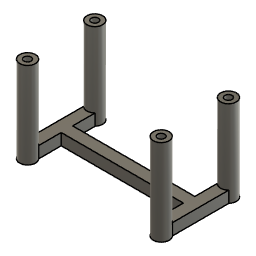
bracketEspHouse (Autodesk Fusion 360 design; units mm, degrees)
Autodesk Fusion 360 part; units mm, degrees
sketch "Schizzo8" plane through (0, 0, 0) normal (0, 1, 0) x (1, 0, 0)
  line L0 (45.3365, 90.3085) -> (91.8565, 90.3085)
  line L1 (91.8565, 90.3085) -> (91.8565, 66.9085)
  line L2 (91.8565, 66.9085) -> (45.3365, 66.9085)
  line L3 (45.3365, 66.9085) -> (45.3365, 90.3085)
  circle A0 centre (45.3365, 90.3085) radius 2.75
  circle A1 centre (91.8565, 90.3085) radius 2.75
  circle A2 centre (91.8565, 66.9085) radius 2.75
  circle A3 centre (45.3365, 66.9085) radius 2.75
  line L4 (45.3365, 90.3085) -> (47.3365, 90.3085)
  line L5 (45.3365, 90.3085) -> (43.3365, 90.3085)
  line L6 (43.3365, 90.3085) -> (43.3365, 66.9085)
  line L7 (47.3365, 90.3085) -> (47.3365, 66.9085)
  line L8 (91.8565, 90.3085) -> (93.8565, 90.3085)
  line L9 (91.8565, 90.3085) -> (89.8565, 90.3085)
  line L10 (89.8565, 90.3085) -> (89.8565, 66.9085)
  line L11 (93.8565, 90.3085) -> (93.8565, 66.9085)
  line L12 (93.8565, 78.6085) -> (93.8565, 80.6085)
  line L13 (93.8565, 78.6085) -> (93.8565, 76.6085)
  line L14 (93.8565, 80.6085) -> (43.3365, 80.6085)
  line L15 (93.8565, 76.6085) -> (43.3365, 76.6085)
  dimension "d71" = 46.52
  dimension "d72" = 23.4
  dimension "d73" = 5.5
  dimension "d74" = 5.5
  dimension "d75" = 5.5
  dimension "d76" = 5.5
  dimension "d77" = 2
  dimension "d78" = 2
  dimension "d79" = 2
  dimension "d80" = 2
  dimension "d81" = 2
  dimension "d82" = 2
  constraint horizontal L0
  constraint vertical L1
  constraint horizontal L2
  constraint vertical L3
  constraint coincident L0.start L3.end
  constraint coincident L0.end L1.start
  constraint coincident L1.end L2.start
  constraint coincident L2.end L3.start
  constraint perpendicular L3 L4
  constraint perpendicular L3 L5
  constraint perpendicular L2 L6
  constraint coincident L2 L7.end
  constraint perpendicular L2 L7
  constraint perpendicular L1 L8
  constraint perpendicular L1 L9
  constraint coincident L2 L10.end
  constraint perpendicular L2 L10
  constraint perpendicular L8 L11
  constraint midpoint L11 L12.start
  constraint parallel L11 L12
  constraint parallel L11 L13
  constraint coincident L6 L14.end
  constraint perpendicular L6 L14
  constraint coincident L6 L15.end
  constraint perpendicular L6 L15
  measures "d71" distance of L0.start L0.end
  measures "d72" distance of L0.start L2.end
  measures "d73" diameter of A0
  measures "d74" diameter of A1
  measures "d75" diameter of A2
  measures "d76" diameter of A3
  measures "d77" distance of L0.start L4.end
  measures "d78" distance of L0.start L5.end
  measures "d79" distance of L0.end L8.end
  measures "d80" distance of L0.end L9.end
  measures "d81" distance of L12.start L12.end
  measures "d82" distance of L12.start L13.end
extrude "Estrusione14" add sketch "Schizzo8" along normal blind 4 contours L3 A0 L7 L14 | L3 A0 L6 L14 | L3 L7 L14 L15 | L3 L6 L14 L15 | L7 L10 L14 L15 | L3 A3 L7 L15 | L3 A3 L6 L15 | L1 A1 L10 L14 | L1 L10 L14 L15 | L1 A1 L11 L14 | L1 A2 L10 L15 | L1 L11 L12 L13 L14 L15 | L1 A2 L11 L15
extrude "Estrusione15" add sketch "Schizzo8" along normal blind 30 contours L0 A0 L4 L5 L6 | L0 L3 A0 L4 L7 | L3 A0 L5 L6 | L0 A0 L7 | L0 A1 L8 L9 L11 | L0 A1 L10 | L0 L1 A1 L9 L10 | L2 L3 A3 L7 | L2 L3 A3 | L1 A1 L8 L11 | L2 A3 L7 | L2 A2 L10 | L1 L2 A2 L10 | L1 L2 A2
hole "Foratura5" at (45.3365, 30, -90.3085) direction (0, -1, 0) diameter 2.5 depth 7 tip angle 118
hole "Foratura6" at (45.3365, 30, -66.9085) direction (0, -1, 0) diameter 2.5 depth 7 tip angle 118
hole "Foratura7" at (91.8565, 30, -66.9085) direction (0, -1, 0) diameter 2.5 depth 7 tip angle 118
hole "Foratura8" at (91.8565, 30, -90.3085) direction (0, -1, 0) diameter 2.5 depth 7 tip angle 118
